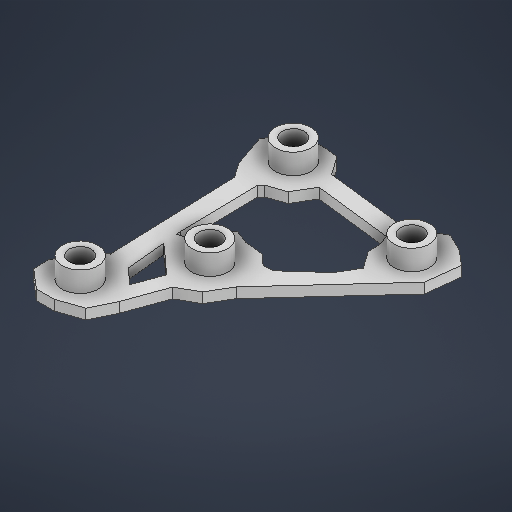
# Autodesk Inventor part: pump holder test
Saved by Autodesk Inventor 2026.1 (Build 301233000, 233)
## iProperties
Created: 2025-11-29
Part Number: pump holder test
Material: Generic
Document SubType Name: Modeling
Designer: maxim
Density: 1 g/cm^3
Appearance: Default
Author: maxim
Autodesk Inventor part; units mm, degrees
ref_plane "YZ Plane" through (0, 0, 0) normal (1, 0, 0) x (0, 1, 0)
ref_plane "XZ Plane" through (0, 0, 0) normal (0, 1, 0) x (-1, 0, 0)
ref_plane "XY Plane" through (0, 0, 0) normal (0, 0, 1) x (1, 0, 0)
sketch "Sketch2" plane through (0, 0, 0) normal (0, 1, 0) x (-1, 0, 0)
  circle A0 centre (126.8658, -60.5977) radius 1.3
  circle A1 centre (126.3381, -85.1348) radius 1.3
  circle A2 centre (120.9816, -69.9614) radius 1.3
  circle A3 centre (109.5738, -82.3141) radius 1.3
  circle A4 centre (126.8658, -60.5977) radius 2.1
  circle A5 centre (120.9816, -69.9614) radius 2.1
  circle A6 centre (126.3381, -85.1348) radius 2.1
  circle A7 centre (109.5738, -82.3141) radius 2.1
  line L0 (130.6426, -58.9167) -> (128.4381, -57.0194)
  line L1 (128.4381, -57.0194) -> (126.3381, -57.0194)
  line L2 (126.3381, -57.0194) -> (123.5561, -57.9681)
  line L3 (123.5561, -57.9681) -> (122.2816, -60.5977)
  line L4 (122.2816, -60.5977) -> (120.6067, -65.2208)
  line L5 (120.6067, -65.2208) -> (118.3664, -66.478)
  line L6 (118.3664, -66.478) -> (116.8823, -68.9845)
  line L7 (116.8823, -68.9845) -> (106.2971, -80.5191)
  line L8 (106.2971, -80.5191) -> (105.8399, -84.4141)
  line L9 (105.8399, -84.4141) -> (107.4814, -85.8269)
  line L10 (107.4814, -85.8269) -> (109.5649, -86.8367)
  line L11 (109.5649, -86.8367) -> (111.3641, -85.8269)
  line L12 (111.3641, -85.8269) -> (113.0075, -84.9046)
  line L13 (113.0075, -84.9046) -> (122.7264, -86.0432)
  line L14 (122.7264, -86.0432) -> (124.2381, -88.177)
  line L15 (124.2381, -88.177) -> (125.7937, -88.3593)
  line L16 (125.7937, -88.3593) -> (128.7617, -88.3593)
  line L17 (128.7617, -88.3593) -> (129.4996, -86.8367)
  line L18 (129.4996, -86.8367) -> (130.6329, -85.5199)
  line L19 (130.6329, -85.5199) -> (129.7559, -82.948)
  line L20 (129.7559, -82.948) -> (129.3357, -81.7158)
  line L21 (129.3357, -81.7158) -> (128.1658, -80.0645)
  line L22 (128.1658, -80.0645) -> (127.6381, -64.9544)
  line L23 (127.6381, -64.9544) -> (129.7126, -62.6938)
  line L24 (129.7126, -62.6938) -> (130.4919, -61.0859)
  line L25 (130.4919, -61.0859) -> (130.7031, -60.6501)
  line L26 (130.7031, -60.6501) -> (130.6426, -58.9167)
  line L27 (125.1674, -64.5771) -> (123.3735, -62.9309)
  line L28 (123.3735, -62.9309) -> (122.2208, -66.1125)
  line L29 (122.2208, -66.1125) -> (124.2158, -67.9433)
  line L30 (124.381, -72.6718) -> (122.5174, -74.7024)
  line L31 (122.5174, -74.7024) -> (120.8801, -74.1092)
  line L32 (120.8801, -74.1092) -> (118.6986, -73.8537)
  line L33 (118.6986, -73.8537) -> (117.4993, -72.753)
  line L34 (117.4993, -72.753) -> (116.3715, -72.7924)
  line L35 (116.3715, -72.7924) -> (112.642, -76.1456)
  line L36 (112.642, -76.1456) -> (111.3266, -78.3671)
  line L37 (111.3266, -78.3671) -> (112.7179, -80.331)
  line L38 (112.7179, -80.331) -> (112.7663, -81.7158)
  line L39 (112.7663, -81.7158) -> (113.1865, -82.948)
  line L40 (113.1865, -82.948) -> (118.6854, -83.5922)
  line L41 (118.6854, -83.5922) -> (122.1722, -84.0006)
  line L42 (122.1722, -84.0006) -> (123.5251, -81.7158)
  line L43 (123.5251, -81.7158) -> (125.5556, -81.0234)
  line L44 (125.5556, -81.0234) -> (125.9926, -80.5472)
  line L45 (125.9926, -80.5472) -> (125.9319, -77.6512)
  line L46 (125.8957, -75.9264) -> (125.7997, -71.3461)
  line L47 (125.8957, -75.9264) -> (125.9319, -77.6512)
  line L48 (124.2158, -67.9433) -> (125.5945, -69.1497)
  line L49 (124.381, -72.6718) -> (124.6636, -71.1574)
  line L50 (124.6636, -71.1574) -> (125.7535, -70.8521)
  line L51 (125.1674, -64.5771) -> (125.5945, -69.1497)
  line L52 (125.7535, -70.8521) -> (125.7997, -71.3461)
  point P0 (0, 0)
  dimension "d1" = 2.6
  dimension "d7" = 2.6
  dimension "d9" = 2.6
  dimension "d11" = 2.6
  dimension "d18" = 0.8
  dimension "d19" = 0.8
  dimension "d20" = 0.8
  dimension "d21" = 0.8
  constraints: 106 end point, 17 parallel, 16 point on line, 9 perpendicular, 8 centre point, 1 horizontal
  measures "d1" diameter of A0
  measures "d7" diameter of A1
  measures "d9" diameter of A2
  measures "d11" diameter of A3
  measures "d18" radial gap between concentric circles of A0 A4
  measures "d19" radial gap between concentric circles of A2 A5
  measures "d20" radial gap between concentric circles of A1 A6
  measures "d21" radial gap between concentric circles of A3 A7
extrude "Extrusion1" add sketch "Sketch2" along normal blind 1.2 contours L26 L25 L24 L23 L22 L21 L20 L19 L18 L17 L16 L15 L14 L13 L12 L11 L10 L9 L8 L7 L6 L5 L4 L3 L2 L1 L0
extrude "Extrusion2" add sketch "Sketch2" along normal blind 3.6 contours A4 | A5 | A6 | A7
body "Solid1"
